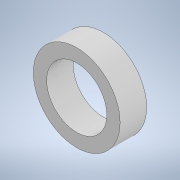
# Autodesk Inventor part: pipeSupportNut
Saved by Autodesk Inventor 2021.1 (Build 251245010, 245A)
## iProperties
Created: 2020-10-20
Part Number: pipeSupportNut
Material: Generic
Document SubType Name: Modeling
Designer: robst
Density: 1 g/cm^3
Appearance: Default
Author: robst
Autodesk Inventor part; units mm, degrees
ref_plane "YZ Plane" through (0, 0, 0) normal (1, 0, 0) x (0, 1, 0)
ref_plane "XZ Plane" through (0, 0, 0) normal (0, 1, 0) x (-1, 0, 0)
ref_plane "XY Plane" through (0, 0, 0) normal (0, 0, 1) x (1, 0, 0)
sketch "Sketch1" plane through (0, 0, 0) normal (0, 0, 1) x (1, 0, 0)
  circle A0 centre (0, 0) radius 7.1926
  circle A1 centre (0, 0) radius 10.3676
  dimension "d0" = 14.3853
  dimension "d1" = 3.175
  constraints: 2 centre point, 2 coincident
  measures "d0" diameter of A0
  measures "d1" radial gap between concentric circles of A1 A0
extrude "Extrusion1" add sketch "Sketch1" against normal blind 6.35
equation "\"d0\" = 0.5 * b1MinorDiameter"
equation "\"d1\" = wallThickness"
equation "\"d2\" = nutWidth"
equation "\"nutWidth\" = 6.35"
equation "\"b1MajorDiameter\" = 31.67634"
equation "\"b1MinorDiameter\" = 28.77058"
equation "\"b1RootRadius\" = 0.18288"
equation "\"wallThickness\" = 3.175"
body "Solid1"
